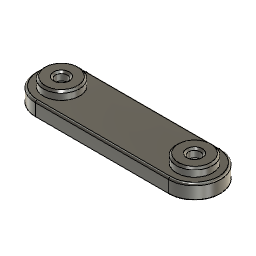
ShaftCap_v5 (Autodesk Fusion 360 design; units mm, degrees)
Autodesk Fusion 360 part; units mm, degrees
sketch "Sketch1" plane through (0, 0, 0) normal (0, 0, 1) x (1, 0, 0) in component "Shaft Cap"
  line L0 (0, 164.1124) -> (0, -164.1124) construction
  line L1 (-160, 0) -> (160, 0) construction
  line L2 (-18, -7) -> (18, -7)
  arc A0 (18, -7) -> (18, 7) centre (18, 0) ccw
  line L3 (18, 7) -> (-18, 7)
  arc A1 (-18, 7) -> (-18, -7) centre (-18, 0) ccw
  line L4 (-18, 0) -> (18, 0) construction
  circle A2 centre (-18, 0) radius 1.625
  circle A3 centre (18, 0) radius 1.625
  circle A4 centre (-18, 0) radius 4.875
  circle A5 centre (18, 0) radius 4.875
  line L5 (-14.6802, 0) -> (-16.3401, 2.875)
  line L6 (-16.3401, 2.875) -> (-19.6599, 2.875)
  line L7 (-19.6599, 2.875) -> (-21.3198, 0)
  line L8 (-21.3198, 0) -> (-19.6599, -2.875)
  line L9 (-19.6599, -2.875) -> (-16.3401, -2.875)
  line L10 (-16.3401, -2.875) -> (-14.6802, 0)
  line L11 (14.6802, 0) -> (16.3401, -2.875)
  line L12 (16.3401, -2.875) -> (19.6599, -2.875)
  line L13 (19.6599, -2.875) -> (21.3198, 0)
  line L14 (21.3198, 0) -> (19.6599, 2.875)
  line L15 (19.6599, 2.875) -> (16.3401, 2.875)
  line L16 (16.3401, 2.875) -> (14.6802, 0)
  point P0 (-18, 0)
  point P1 (18, 0)
  dimension "d1" = 14
  dimension "d2" = 36
  dimension "d3" = 3.25
  dimension "d4" = 9.75
  dimension "d5" = 5.75
  constraint midpoint origin L1
  constraint midpoint origin L0
  constraint horizontal L1
  constraint vertical L0
  constraint tangent L2 A0
  constraint tangent A0 L3
  constraint parallel L2 L3
  constraint tangent L3 A1
  constraint tangent L2 A1
  constraint coincident L1 P1
  constraint perpendicular L0 L4
  constraint midpoint L4 origin
  constraint concentric A1 A2
  constraint concentric A0 A3
  constraint equal A2 A3
  constraint concentric A2 A4
  constraint concentric A0 A5
  constraint equal A4 A5
  constraint coincident P0 A1.centre
  constraint coincident L4 L5.start
  constraint coincident P1 A0.centre
  constraint coincident L4 L11.start
  constraint collinear L6 L15
  measures "d1" distance of L2 L3
  measures "d2" distance of P0 P1
  measures "d3" diameter of A2
  measures "d4" diameter of A4
  measures "d5" distance of L6 L9
extrude "Extrude1" add sketch "Sketch1" against normal blind 4 contours L2 A0 L3 A1 | A4 | A5 | L5 L6 L7 L8 L9 L10 | L11 L12 L13 L14 L15 L16 in component "Shaft Cap"
extrude "Extrude2" add sketch "Sketch1" along normal blind 2.2 contours A4 | A5 | L5 L6 L7 L8 L9 L10 | L11 L12 L13 L14 L15 L16 in component "Shaft Cap"
extrude "Extrude3" cut sketch "Sketch1" along normal blind 4 from surface at -4 contours L5 L6 L7 L8 L9 L10 | L11 L12 L13 L14 L15 L16 in component "Shaft Cap"
fillet "Fillet1" radius 0.5 4 edges at (-25, 0, 0) (0, -7, 0) (25, 0, 0) (0, 7, 0) in component "Shaft Cap"
fillet "Fillet1" radius 0.25 4 edges at (-25, 0, -4) (0, 7, -4) (25, 0, -4) (0, -7, -4) in component "Shaft Cap"
fillet "Fillet2" radius 0.25 12 edges at (-18, -2.875, -4) (-20.4898, -1.4375, -4) (-20.4898, 1.4375, -4) (-18, 2.875, -4) (-15.5102, 1.4375, -4) (-15.5102, -1.4375, -4) (18, -2.875, -4) (15.5102, -1.4375, -4) (15.5102, 1.4375, -4) (18, 2.875, -4) (20.4898, 1.4375, -4) (20.4898, -1.4375, -4) in component "Shaft Cap"
chamfer "Chamfer1" distance 0.5 angle 45 2 edges at (13.4549, -1.7629, 2.2) (-22.5451, -1.7629, 2.2) in component "Shaft Cap"
chamfer "Chamfer1" distance 0.5 angle 45 2 edges at (-19.515, 0.5876, 2.2) (16.485, 0.5876, 2.2) in component "Shaft Cap"
component "Shaft Cap" placed x (1, 0, 0) y (0, 1, 0) z (0, 0, 1) at (0, 0, 0)
